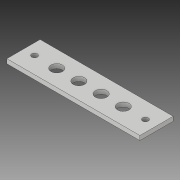
# Autodesk Inventor part: Vial_Plate
Saved by Autodesk Inventor 2019 (Build 230136000, 136)
## iProperties
Created: 2021-08-02
Part Number: Vial_Plate
Material: Generic
Document SubType Name: Modeling
Designer: devon
Density: 1 g/cm^3
Appearance: Default
Author: devon
Autodesk Inventor part; units mm, degrees
ref_plane "YZ Plane" through (0, 0, 0) normal (1, 0, 0) x (0, 1, 0)
ref_plane "XZ Plane" through (0, 0, 0) normal (0, 1, 0) x (-1, 0, 0)
ref_plane "XY Plane" through (0, 0, 0) normal (0, 0, 1) x (1, 0, 0)
sketch "Sketch1" plane through (0, 0, 0) normal (0, 1, 0) x (-1, 0, 0)
  line L0 (76.2, 19.05) -> (-76.2, 19.05)
  line L1 (-76.2, 19.05) -> (-76.2, -19.05)
  line L2 (-76.2, -19.05) -> (76.2, -19.05)
  line L3 (76.2, -19.05) -> (76.2, 19.05)
  line L4 (76.2, 19.05) -> (-76.2, -19.05) construction
  line L5 (-76.2, 19.05) -> (76.2, -19.05) construction
  point P0 (0, 0)
  dimension "d0" = 152.4
  dimension "d1" = 38.1
  constraints: 12 end point, 2 midpoint, 2 parallel, 1 horizontal, 1 perpendicular
  measures "d0" distance of L1.end L2.end
  measures "d1" distance of L2.end L0.start
extrude "Extrusion1" add sketch "Sketch1" along normal blind 5
sketch "Sketch2" plane through (0, 5, 0) normal (0, 1, 0) x (1, 0, 0)
  circle A0 centre (-38.1, 0) radius 6.6
  circle A1 centre (-12.7, 0) radius 6.6
  circle A2 centre (12.7, 0) radius 6.6
  circle A3 centre (38.1, 0) radius 6.6
  line L0 (-76.2, 19.05) -> (-76.2, -19.05) projected
  line L1 (76.2, -19.05) -> (76.2, 19.05) projected
  circle A4 centre (-63.5, 0) radius 3.3
  circle A5 centre (63.5, 0) radius 3.3
  point P0 (0, 0)
  dimension "d4" = 13.2
  dimension "d5" = 13.2
  dimension "d6" = 13.2
  dimension "d7" = 13.2
  dimension "d8" = 25.4
  dimension "d9" = 25.4
  dimension "d10" = 25.4
  dimension "d12" = 38.1
  dimension "d13" = 6.6
  dimension "d14" = 6.6
  dimension "d15" = 12.7
  dimension "d16" = 12.7
  constraints: 6 centre point
  measures "d4" diameter of A0
  measures "d5" diameter of A1
  measures "d6" diameter of A2
  measures "d7" diameter of A3
  measures "d8" distance of A1.centre A0.centre
  measures "d9" distance of A3.centre A2.centre
  measures "d10" distance of A1.centre A2.centre
  measures "d12" distance from line of L1 A3.centre
  measures "d13" diameter of A4
  measures "d14" diameter of A5
  measures "d15" distance from line of L0 A4.centre
  measures "d16" distance from line of L1 A5.centre
extrude "Extrusion2" cut sketch "Sketch2" against normal up to next
body "Solid1"
